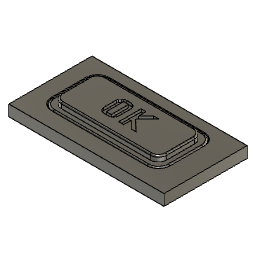
Week 3 HW Button (Autodesk Fusion 360 design; units mm, degrees)
Autodesk Fusion 360 part; units mm, degrees
sketch "Sketch1" plane through (0, 0, 0) normal (0, 0, 1) x (1, 0, 0)
  line L0 (40, -30) -> (230, -30)
  line L1 (230, -30) -> (230, -110)
  line L2 (230, -110) -> (40, -110)
  line L3 (40, -110) -> (40, -30)
  line L4 (30, -20) -> (240, -20)
  line L5 (240, -20) -> (240, -120)
  line L6 (240, -120) -> (30, -120)
  line L7 (30, -120) -> (30, -20)
  line L8 (40, -30) -> (230, -110)
  line L9 (230, -30) -> (40, -110)
  line L10 (241, -121) -> (29, -121)
  line L11 (29, -121) -> (29, -19)
  line L12 (29, -19) -> (241, -19)
  line L13 (241, -19) -> (241, -121)
  line L14 (241, -121) -> (29, -19) construction
  line L15 (29, -121) -> (241, -19) construction
  line L16 (0, 0) -> (280, 0)
  line L17 (280, 0) -> (280, -150)
  line L18 (280, -150) -> (0, -150)
  line L19 (0, -150) -> (0, 0)
  point P0 (135, -70)
  constraint horizontal L0
  constraint vertical L1
  constraint horizontal L2
  constraint vertical L3
  constraint horizontal L4
  constraint vertical L5
  constraint horizontal L6
  constraint vertical L7
  constraint horizontal L10
  constraint perpendicular L10 L11
  constraint parallel L10 L12
  constraint parallel L11 L13
  constraint coincident L14 P0
  constraint coincident L15 P0
  constraint midpoint L8 P0
  constraint horizontal L16
  constraint vertical L17
  constraint horizontal L18
  constraint vertical L19
  constraint coincident L16.start L19.end
extrude "Extrude3" add sketch "Sketch1" against normal blind 20 contours L16 L17 L18 L19 makes body 1
extrude "Extrude1" add sketch "Sketch1" against normal blind 20 separate body contours L3 L8 L9 | L0 L8 L9 | L1 L8 L9 | L2 L8 L9 | L4 L5 L6 L7 makes body 2
extrude "Extrude2" add sketch "Sketch1" along normal blind 10 contours L3 L8 L9 | L0 L8 L9 | L1 L8 L9 | L2 L8 L9 bodies 2
fillet "Fillet1" radius 15 4 edges at (40, -110, 5) (40, -30, 5) (230, -30, 5) (230, -110, 5) on bodies 2
fillet "Fillet1" radius 20 4 edges at (30, -120, -10) (30, -20, -10) (240, -20, -10) (240, -120, -10) on bodies 2
fillet "Fillet2" radius 2.5 16 edges at (225.6066, -34.3934, 10) (135, -30, 10) (44.3934, -34.3934, 10) (40, -70, 10) (44.3934, -105.6066, 10) (135, -110, 10) (225.6066, -105.6066, 10) (230, -70, 10) (30, -70, 0) (35.8579, -25.8579, 0) (135, -20, 0) (234.1421, -25.8579, 0) (240, -70, 0) (234.1421, -114.1421, 0) (135, -120, 0) (35.8579, -114.1421, 0) on bodies 2
fillet "Fillet3" radius 20 4 edges at (29, -19, -10) (241, -19, -10) (241, -121, -10) (29, -121, -10) on bodies 1
fillet "Fillet4" radius 1 8 edges at (235.1421, -115.1421, 0) (241, -70, 0) (235.1421, -24.8579, 0) (135, -19, 0) (34.8579, -24.8579, 0) (29, -70, 0) (34.8579, -115.1421, 0) (135, -121, 0) on bodies 1
sketch "Sketch2" plane through (0, 0, 10) normal (0, 0, 1) x (-1, 0, 0)
  arc A0 (-227.5, 45) -> (-215, 32.5) centre (-215, 45) ccw
  line L0 (-215, 32.5) -> (-55, 32.5)
  arc A1 (-55, 32.5) -> (-42.5, 45) centre (-55, 45) ccw
  line L1 (-42.5, 45) -> (-42.5, 95)
  arc A2 (-42.5, 95) -> (-55, 107.5) centre (-55, 95) ccw
  line L2 (-55, 107.5) -> (-215, 107.5)
  arc A3 (-215, 107.5) -> (-227.5, 95) centre (-215, 95) ccw
  line L3 (-227.5, 95) -> (-227.5, 45)
  line L4 (-110.0488, 48.1218) -> (-118.633, 48.1218)
  spline S0 degree 3 poles (-118.633, 48.1218) (-119.851, 48.1218) (-120.9965, 48.3611) (-122.084, 48.8469) knots 0 0 0 0 1 1 1 1
  spline S1 degree 3 poles (-122.084, 48.8469) (-123.1861, 49.3254) (-124.1576, 49.9924) (-125.0131, 50.8479) knots 0 0 0 0 1 1 1 1
  spline S2 degree 3 poles (-125.0131, 50.8479) (-125.8614, 51.6962) (-126.5356, 52.6604) (-127.0431, 53.748) knots 0 0 0 0 1 1 1 1
  spline S3 degree 3 poles (-127.0431, 53.748) (-127.5434, 54.85) (-127.7972, 56.0173) (-127.7972, 57.257) knots 0 0 0 0 1 1 1 1
  line L5 (-127.7972, 57.257) -> (-127.7972, 79.4715)
  spline S4 degree 3 poles (-127.7972, 79.4715) (-127.7972, 80.6315) (-127.5507, 81.748) (-127.0722, 82.8356) knots 0 0 0 0 1 1 1 1
  spline S5 degree 3 poles (-127.0722, 82.8356) (-126.5864, 83.9376) (-125.9266, 84.9091) (-125.1001, 85.7646) knots 0 0 0 0 1 1 1 1
  spline S6 degree 3 poles (-125.1001, 85.7646) (-124.2663, 86.6129) (-123.2876, 87.3017) (-122.171, 87.8237) knots 0 0 0 0 1 1 1 1
  spline S7 degree 3 poles (-122.171, 87.8237) (-121.069, 88.3457) (-119.8873, 88.6067) (-118.633, 88.6067) knots 0 0 0 0 1 1 1 1
  line L6 (-118.633, 88.6067) -> (-110.0488, 88.6067)
  spline S8 degree 3 poles (-110.0488, 88.6067) (-108.7873, 88.6067) (-107.5982, 88.3457) (-106.4817, 87.8237) knots 0 0 0 0 1 1 1 1
  spline S9 degree 3 poles (-106.4817, 87.8237) (-105.358, 87.3017) (-104.3792, 86.6129) (-103.5527, 85.7646) knots 0 0 0 0 1 1 1 1
  spline S10 degree 3 poles (-103.5527, 85.7646) (-102.7406, 84.9091) (-102.0809, 83.9376) (-101.5806, 82.8356) knots 0 0 0 0 1 1 1 1
  spline S11 degree 3 poles (-101.5806, 82.8356) (-101.0949, 81.748) (-100.8556, 80.6315) (-100.8556, 79.4715) knots 0 0 0 0 1 1 1 1
  line L7 (-100.8556, 79.4715) -> (-100.8556, 57.257)
  spline S12 degree 3 poles (-100.8556, 57.257) (-100.8556, 56.0173) (-101.1021, 54.85) (-101.6096, 53.748) knots 0 0 0 0 1 1 1 1
  spline S13 degree 3 poles (-101.6096, 53.748) (-102.1099, 52.6604) (-102.7841, 51.6962) (-103.6397, 50.8479) knots 0 0 0 0 1 1 1 1
  spline S14 degree 3 poles (-103.6397, 50.8479) (-104.4879, 49.9924) (-105.4522, 49.3254) (-106.5397, 48.8469) knots 0 0 0 0 1 1 1 1
  spline S15 degree 3 poles (-106.5397, 48.8469) (-107.6417, 48.3611) (-108.809, 48.1218) (-110.0488, 48.1218) knots 0 0 0 0 1 1 1 1
  line L8 (-118.836, 52.6459) -> (-109.8168, 52.6459)
  line L9 (-109.8168, 52.6459) -> (-109.8168, 84.1116)
  line L10 (-109.8168, 84.1116) -> (-118.836, 84.1116)
  line L11 (-118.836, 84.1116) -> (-118.836, 52.6459)
  line L12 (-159.2957, 88.6067) -> (-145.8104, 75.0054)
  line L13 (-145.8104, 75.0054) -> (-145.8104, 88.6067)
  line L14 (-145.8104, 88.6067) -> (-136.8492, 88.6067)
  line L15 (-136.8492, 88.6067) -> (-136.8492, 48.1219)
  line L16 (-136.8492, 48.1219) -> (-145.8104, 48.1219)
  line L17 (-145.8104, 48.1219) -> (-145.8104, 61.7811)
  line L18 (-145.8104, 61.7811) -> (-159.2957, 48.1219)
  line L19 (-159.2957, 48.1219) -> (-168.3149, 48.1219)
  line L20 (-168.3149, 48.1219) -> (-147.8695, 69.2343)
  line L21 (-147.8695, 69.2343) -> (-168.3149, 88.6067)
  line L22 (-168.3149, 88.6067) -> (-159.2957, 88.6067)
extrude "Extrude4" cut sketch "Sketch2" against normal blind 5 contours L4 S0 S1 S2 S3 L5 S4 S5 S6 S7 L6 S8 S9 S10 S11 L7 S12 S13 S14 S15 | L12 L13 L14 L15 L16 L17 L18 L19 L20 L21 L22 bodies 2
